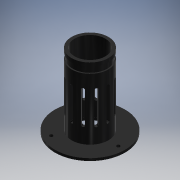
# Autodesk Inventor part: ValveStem
Saved by Autodesk Inventor 2017 (Build 210142000, 142)
## iProperties
Created: 2017-03-13
Part Number: ValveStem
Material: Acetal Resin, Black
Document SubType Name: Modeling
Designer: Joseph
Density: 1.425 g/cm^3
Appearance: Smooth - Black
Mass: 44.3835 g
Surface Area: 242.034 cm^2
Volume: 31.1463 cm^3
Author: Joseph
Autodesk Inventor part; units mm, degrees
ref_plane "YZ Plane" through (0, 0, 0) normal (1, 0, 0) x (0, 1, 0)
ref_plane "XZ Plane" through (0, 0, 0) normal (0, 1, 0) x (-1, 0, 0)
sketch "Sketch1" plane through (0, 0, 0) normal (0, 1, 0) x (-1, 0, 0)
  circle A0 centre (0, 0) radius 36.195
  dimension "d0" = 72.39
  constraints: 1 centre point, 1 coincident
  measures "d0" diameter of A0
extrude "Extrusion1" add sketch "Sketch1" along normal blind 2.54
sketch "Sketch2" plane through (0, 2.54, 0) normal (0, 1, 0) x (1, 0, 0)
  circle A0 centre (0, 0) radius 15.9004
  circle A1 centre (0, 0) radius 19.05
  dimension "d3" = 31.8008
  dimension "d4" = 38.1
  constraints: 2 centre point, 2 coincident
  measures "d3" diameter of A0
  measures "d4" diameter of A1
extrude "Extrusion2" add sketch "Sketch2" along normal blind 73.66
ref_plane "Work Plane1" through (0, 2.54, 19.05) normal (0, 0, 1) x (1, 0, 0)
sketch "Sketch3" plane through (0, 2.54, 19.05) normal (0, 0, 1) x (1, 0, 0)
  line L0 (-1.8571, 16.835) -> (-1.8571, 48.66)
  line L1 (1.3179, 16.835) -> (1.3179, 48.66)
  arc A0 (1.3179, 48.66) -> (-1.8571, 48.66) centre (-0.2696, 48.66) ccw
  arc A1 (-1.8571, 16.835) -> (1.3179, 16.835) centre (-0.2696, 16.835) ccw
  line L2 (-15.9004, 73.66) -> (15.9004, 73.66) projected
  point P0 (0, -2.54)
  dimension "d7" = 3.175
  dimension "d8" = 35
  dimension "d9" = 25
  constraints: 4 end point, 4 point on circle, 4 tangent, 2 centre point, 2 vertical
  measures "d7" distance between parallel lines of L1 L0
  measures "d9" distance from line of L2 A0.centre
extrude "Extrusion3" cut sketch "Sketch3" against normal blind 10
pattern_circular "Circular Pattern1" count 12 over 360 about axis through (0, 2.54, 0) along (0, 1, 0) of "Extrusion3"
sketch "Sketch4" plane through (0, 2.54, 0) normal (0, 1, 0) x (1, 0, 0)
  circle A0 centre (0, 0) radius 15.7607
  dimension "d15" = 31.5214
  constraints: 1 centre point, 1 coincident
  measures "d15" diameter of A0
extrude "Extrusion4" cut sketch "Sketch4" against normal blind 50
sketch "Sketch5" plane through (0, 0, 0) normal (0, 0, 1) x (1, 0, 0)
  line L0 (17.78, 66.04) -> (19.05, 66.04)
  line L1 (19.05, 66.04) -> (19.05, 72.39)
  line L2 (19.05, 72.39) -> (17.78, 72.39)
  line L3 (17.78, 72.39) -> (17.78, 66.04)
  line L4 (-15.9004, 76.2) -> (15.9004, 76.2) projected
  line L5 (0, -15.508) -> (0, 93.048) projected
  point P0 (0, 0)
  dimension "d18" = 6.35
  dimension "d19" = 3.81
  dimension "d21" = 19.05
  dimension "d22" = 1.27
  constraints: 8 end point, 2 parallel, 1 horizontal, 1 perpendicular
  measures "d18" distance between parallel lines of L0 L2
  measures "d19" distance between parallel lines of L4 L2
  measures "d21" distance from line of point (0, 0) L1
  measures "d22" distance of L1.end L2.end
revolve "Revolution1" cut sketch "Sketch5" angle 360 about axis through (0, -10, 0) along (0, 1, 0)
sketch "Sketch6" plane through (0, 0, 0) normal (0, -1, 0) x (1, 0, 0)
  line L0 (0, 0) -> (29.3624, 0)
  dimension "d24" = 29.3624
  constraints: 2 end point, 1 horizontal
  measures "d24" distance of L0.start L0.end
hole "Hole1" at (29.3624, 0, 0) direction (0, 1, 0) diameter 3.5052 end through all
pattern_circular "Circular Pattern2" count 3 over 360 about axis through (0, 2.54, 0) along (0, 1, 0) of "Hole1"
body "Solid1"
